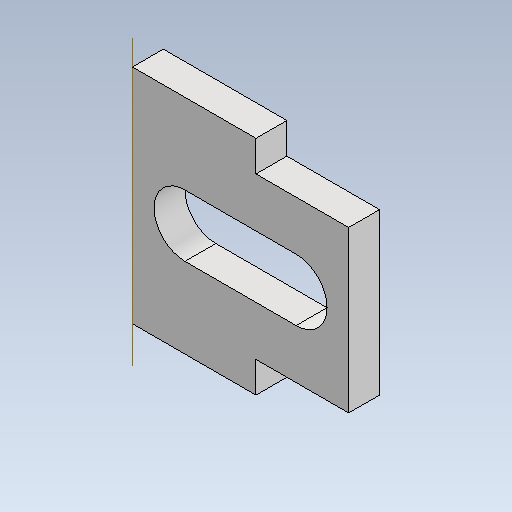
# Autodesk Inventor part: r-support
Saved by Autodesk Inventor 2025 (Build 290162000, 162)
## iProperties
Created: 2025-08-21
Part Number: r-support
Material: Generic
Document SubType Name: Modeling
Designer: HP
Density: 1 g/cm^3
Appearance: Default
Author: HP
Autodesk Inventor part; units mm, degrees
ref_plane "YZ Plane" through (0, 0, 0) normal (1, 0, 0) x (0, 1, 0)
ref_plane "XZ Plane" through (0, 0, 0) normal (0, 1, 0) x (-1, 0, 0)
ref_plane "XY Plane" through (0, 0, 0) normal (0, 0, 1) x (1, 0, 0)
sketch "Sketch1" plane through (0, 0, 0) normal (0, 0, 1) x (1, 0, 0)
  line L0 (-17.5, -18) -> (17.5, -18)
  line L1 (17.5, -18) -> (17.5, 18)
  line L2 (17.5, 18) -> (-17.5, 18)
  line L3 (-17.5, 18) -> (-17.5, -18)
  line L4 (-17.5, -18) -> (17.5, 18) construction
  line L5 (17.5, -18) -> (-17.5, 18) construction
  line L6 (17.5, 18) -> (2.5, 18)
  line L7 (2.5, 18) -> (2.5, 13)
  line L8 (2.5, 13) -> (17.5, 13)
  line L9 (17.5, 13) -> (17.5, 18)
  line L10 (17.5, -18) -> (2.5, -18)
  line L11 (2.5, -18) -> (2.5, -13)
  line L12 (2.5, -13) -> (17.5, -13)
  line L13 (17.5, -13) -> (17.5, -18)
  line L14 (-9, 0) -> (9, 0) construction
  line L15 (-9, -5) -> (9, -5)
  line L16 (9, 5) -> (-9, 5)
  arc A0 (-9, 5) -> (-9, -5) centre (-9, 0) ccw
  arc A1 (9, -5) -> (9, 5) centre (9, 0) ccw
  point P0 (0, 0)
  point P1 (2.5, -18)
  point P2 (17.5, 13)
  point P3 (0, 0)
  point P4 (-17.5, 0)
  dimension "d0" = 36
  dimension "d1" = 35
  dimension "d2" = 5
  dimension "d3" = 5
  dimension "d4" = 20
  dimension "d7" = 10
  dimension "d8" = 18
  constraints: 36 end point, 7 parallel, 4 horizontal, 4 midpoint, 4 point on circle, 4 tangent, 3 perpendicular, 2 centre point, 1 coincident, 1 collinear, 1 horizontal alignment
  measures "d0" distance between parallel lines of L0 L2
  measures "d1" distance between parallel lines of L1 L3
  measures "d2" distance between parallel lines of L8 L2
  measures "d3" distance between parallel lines of L0 L12
  measures "d4" distance between parallel lines of L3 L7
  measures "d7" diameter of A1
  measures "d8" distance of L14.start L14.end
extrude "Extrusion1" add sketch "Sketch1" along normal blind 5 contours L3 L2 L7 L8 L1 L12 L11 L0
equation "\"d3\" = d2"
body "Solid1"
